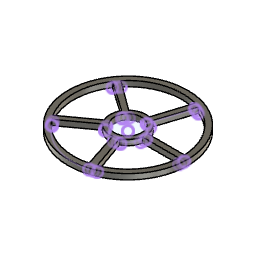
wheel_model v2 (Autodesk Fusion 360 design; units mm, degrees)
Autodesk Fusion 360 part; units mm, degrees
sketch "Sketch1" plane through (0, 0, 0) normal (0, 0, 1) x (1, 0, 0)
  circle A0 centre (0, 0) radius 25
  circle A1 centre (0, 0) radius 30
  circle A2 centre (0, 0) radius 100
  circle A3 centre (0, 0) radius 110
  line L0 (0, 0) -> (9.2705, 28.5317)
  line L1 (0, 0) -> (30, 0) construction
  line L2 (0, 0) -> (5.2094, 29.5442)
  line L3 (0, 0) -> (70, 0) construction
  line L4 (9.2705, 28.5317) -> (30.9017, 95.1057)
  line L5 (5.2094, 29.5442) -> (26.1292, 96.526)
  line L6 (0, 0) -> (-24.2705, 17.6336)
  line L7 (0, 0) -> (30, 0) construction
  line L8 (0, 0) -> (-25.9808, 15)
  line L9 (0, 0) -> (30, 0) construction
  line L10 (-24.2705, 17.6336) -> (-80.6713, 59.0943)
  line L11 (-25.9808, 15) -> (-83.4848, 55.048)
  line L12 (0, 0) -> (-24.2705, -17.6336)
  line L13 (0, 0) -> (30, 0) construction
  line L14 (0, 0) -> (-22.2943, -20.0739)
  line L15 (0, 0) -> (30, 0) construction
  line L16 (-24.2705, -17.6336) -> (-80.9017, -58.7785)
  line L17 (-22.2943, -20.0739) -> (-79.0187, -61.2866)
  line L18 (0, 0) -> (-30, 0) construction
  line L19 (0, 0) -> (9.2705, -28.5317)
  line L20 (0, 0) -> (30, 0) construction
  line L21 (0, 0) -> (13.1511, -26.9638)
  line L22 (0, 0) -> (30, 0) construction
  line L23 (9.2705, -28.5317) -> (30.9017, -95.1057)
  line L24 (13.1511, -26.9638) -> (36.5741, -93.0717)
  line L25 (30, 0) -> (100, 0)
  line L26 (29.7329, 3.994) -> (99.9202, 3.994)
  dimension "d1" = 50
  dimension "d2" = 60
  dimension "d5" = 200
  dimension "d6" = 220
  dimension "d7" = 30
  dimension "d8" = 72
  dimension "d9" = 80
  dimension "d10" = 30
  dimension "d12" = 70.1726
  dimension "d13" = 144
  dimension "d14" = 30
  dimension "d15" = 150
  dimension "d16" = 30
  dimension "d17" = 70.0003
  dimension "d18" = 70.0754
  dimension "d19" = 144
  dimension "d20" = 30
  dimension "d21" = 138
  dimension "d22" = 30
  dimension "d25" = 72
  dimension "d26" = 30
  dimension "d27" = 64
  dimension "d28" = 30
  dimension "d29" = 70.1347
  dimension "d30" = 70.1873
  constraint coincident A0.centre A1.centre
  constraint concentric A0 A2
  constraint concentric A0 A3
  constraint horizontal L1
  constraint horizontal L3
  constraint coincident A2 L4.end
  constraint parallel L0 L4
  constraint coincident A2 L5.end
  constraint horizontal L7
  constraint horizontal L9
  constraint coincident A2 L10.end
  constraint coincident A2 L11.end
  constraint horizontal L13
  constraint horizontal L15
  constraint coincident A2 L16.end
  constraint parallel L12 L16
  constraint coincident A2 L17.end
  constraint parallel L16 L17
  constraint horizontal L18
  constraint horizontal L20
  constraint horizontal L22
  constraint coincident A2 L23.end
  constraint parallel L19 L23
  constraint coincident A2 L24.end
  constraint coincident A2 L25.end
  constraint parallel L3 L25
  constraint coincident A1 L26.start
  constraint coincident A2 L26.end
  constraint parallel L9 L26
  measures "d1" diameter of A0
  measures "d2" diameter of A1
  measures "d5" diameter of A2
  measures "d6" diameter of A3
  measures "d7" distance of A0.centre L0.end
  measures "d8" angle of L0 L1
  measures "d9" angle of L2 L3
  measures "d10" distance of A0.centre L2.end
  measures "d12" distance of L2.end L5.end
  measures "d13" angle of L6 L7
  measures "d14" distance of A0.centre L6.end
  measures "d15" angle of L8 L9
  measures "d16" distance of A0.centre L8.end
  measures "d17" distance of L6.end L10.end
  measures "d18" distance of L8.end L11.end
  measures "d19" angle of L12 L13
  measures "d20" distance of A0.centre L12.end
  measures "d21" angle of L14 L15
  measures "d22" distance of A0.centre L14.end
  measures "d25" angle of L19 L20
  measures "d26" distance of A0.centre L19.end
  measures "d27" angle of L21 L22
  measures "d28" distance of A0.centre L21.end
  measures "d29" distance of L21.end L24.end
  measures "d30" distance of L26.start L26.end
extrude "Extrude1" add sketch "Sketch1" along normal blind 10 contours A0 A1 L0 L21 | A0 A1 L0 L2 | A0 A1 L19 L21 | A0 A1 L2 L6 | A1 A2 L4 L5 | A0 A1 L14 L19 | A1 A2 L23 L24 | A0 A1 L6 L8 | A0 A1 L8 L12 | A0 A1 L12 L14 | A1 A2 L25 L26 | A1 A2 L10 L11 | A1 A2 L16 L17 | A3
sketch "Sketch2" plane through (0, 0, 0) normal (0, 0, 1) x (1, 0, 0)
  point P0 (-24.2705, -17.6336)
  point P1 (-22.2943, -20.0739)
  point P2 (9.2705, -28.5317)
  point P3 (13.1511, -26.9638)
  point P4 (30, 0)
  point P5 (29.7329, 3.994)
  point P6 (5.2094, 29.5442)
  point P7 (9.2705, 28.5317)
  point P8 (-25.9808, 15)
  point P9 (-24.2705, 17.6336)
  point P10 (30.9017, -95.1057)
  point P11 (36.5741, -93.0717)
  point P12 (100, 0)
  point P13 (99.9202, 3.994)
  point P14 (-80.9017, -58.7785)
  point P15 (-79.0187, -61.2866)
  point P16 (-83.4848, 55.048)
  point P17 (-80.6713, 59.0943)
  point P18 (26.1292, 96.526)
  point P19 (30.9017, 95.1057)
move_face "OffsetFaces1" offset 6 1 faces at (16.4809, 50.723, 3.3333)
sketch "Sketch3" plane through (0, 0, 0) normal (0, 0, 1) x (1, 0, 0)
  line L0 (26.1292, 96.526) -> (5.2094, 29.5442)
  point P0 (36.5524, 93.0802)
move_face "OffsetFaces2" offset -1 1 faces at (12.1827, 51.8715, 3.3333)
move_face "OffsetFaces3" offset 6 1 faces at (53.3333, 0, 3.3333)
move_face "OffsetFaces4" offset 6 3 faces at (23.6913, -72.9143, 6.6667) (-62.0246, -45.0635, 6.6667) (-43.0708, 31.4538, 3.3333)
sketch "Sketch4" plane through (0, 0, 0) normal (0, 0, 1) x (1, 0, 0)
  circle A0 centre (0, 0) radius 25
  arc A1 (-79.0187, -61.2866) -> (25.1397, -96.7884) centre (0, 0) ccw
  point P0 (-76.9805, 63.8279)
  point P1 (-83.4848, 55.048)
  point P2 (-79.0187, -61.2866)
  point P3 (-84.2827, -53.8185)
  point P4 (36.5741, -93.0717)
  point P5 (25.1397, -96.7884)
  point P6 (99.9202, 3.994)
  point P7 (99.8198, -6)
  point P8 (36.5524, 93.0802)
  point P9 (26.1292, 96.526)
  point P10 (13.1511, -26.9638)
  point P11 (3.3769, -29.8093)
  point P12 (-22.2943, -20.0739)
  point P13 (-27.3069, -12.4232)
  point P14 (-20.2559, 22.1291)
  point P15 (-25.9808, 15)
  point P16 (14.7895, 26.1011)
  point P17 (5.2094, 29.5442)
  point P18 (29.7329, 3.994)
  point P19 (29.3939, -6)
move_face "OffsetFaces5" offset 3 1 faces at (28.7596, -8.5372, 3.3333)
move_face "OffsetFaces6" offset 3 1 faces at (17.021, 24.704, 3.3333)
move_face "OffsetFaces7" offset 3 1 faces at (-19.2352, 23.0219, 3.3333)
move_face "OffsetFaces8" offset 3 2 faces at (0.6681, -29.9926, 3.3333) (-28.3182, -9.9036, 3.3333)
